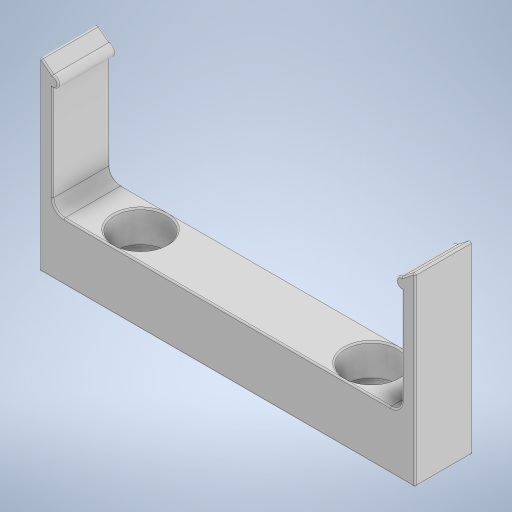
# Autodesk Inventor part: Top bot holder
Saved by Autodesk Inventor 2024 (Build 280153000, 153)
## iProperties
Created: 2024-04-04
Part Number: Top bot holder
Material: Generic
Document SubType Name: Modeling
Designer: jens1
Density: 1 g/cm^3
Appearance: Default
Author: jens1
## iProperties of the stored document Top bot holder_3DPrint.ipt
Created: 2024-04-04
Part Number: Top bot holder_3DPrint
Material: Generic
Document SubType Name: Modeling
Designer: jens1
Density: 1 g/cm^3
Appearance: Default
Author: jens1
Autodesk Inventor part; units mm, degrees
ref_plane "YZ Plane" through (0, 0, 0) normal (1, 0, 0) x (0, 1, 0)
ref_plane "XZ Plane" through (0, 0, 0) normal (0, 1, 0) x (-1, 0, 0)
ref_plane "XY Plane" through (0, 0, 0) normal (0, 0, 1) x (1, 0, 0)
sketch "Sketch1" plane through (0, 0, 0) normal (0, 0, 1) x (1, 0, 0)
  line L0 (0, 0) -> (65, 0)
  line L1 (65, 0) -> (65, 10)
  line L2 (65, 10) -> (0, 10)
  line L3 (0, 10) -> (0, 0)
  line L4 (0, 10) -> (2.25, 10)
  line L5 (2.25, 10) -> (2.25, 30.5)
  line L6 (2.25, 30.5) -> (0, 30.5)
  line L7 (0, 30.5) -> (0, 10)
  circle A0 centre (2.25, 29.5) radius 1
  line L8 (65, 10) -> (62.75, 10)
  line L9 (62.75, 10) -> (62.75, 30.5)
  line L10 (62.75, 30.5) -> (65, 30.5)
  line L11 (65, 30.5) -> (65, 10)
  circle A1 centre (62.75, 29.5) radius 1
  line L12 (0, 30.5) -> (2.25, 30.5)
  line L13 (2.25, 30.5) -> (2.25, 32.25)
  line L14 (2.25, 32.25) -> (0, 32.25)
  line L15 (0, 32.25) -> (0, 30.5)
  line L16 (62.75, 30.5) -> (65, 30.5)
  line L17 (65, 30.5) -> (65, 32.25)
  line L18 (65, 32.25) -> (62.75, 32.25)
  line L19 (62.75, 32.25) -> (62.75, 30.5)
  line L20 (0, 32.25) -> (2.25, 30.5)
  line L21 (62.75, 30.5) -> (65, 32.25)
  point P0 (62.75, 28.5)
  point P1 (2.25, 10)
  point P2 (2.25, 28.5)
  dimension "d4" = 2
  dimension "d7" = 2
  dimension "d0" = 65
  dimension "d1" = 10
  dimension "d2" = 2.25
  dimension "d3" = 20.5
  dimension "d5" = 2.25
  dimension "d6" = 20.5
  dimension "d31" = 2.25
  dimension "d32" = 1.75
  dimension "d33" = 2.25
  dimension "d34" = 1.75
  constraints: 44 end point, 10 parallel, 5 horizontal, 5 perpendicular, 2 point on line, 6 other
  measures "d0" distance of L2.end L1.end
  measures "d1" distance of L1.end L0.end
  measures "d2" distance of L6.end L5.end
  measures "d3" distance of L5.end L4.end
  measures "d5" distance of L9.end L10.end
  measures "d6" distance of L8.end L9.end
  measures "d31" distance of L14.end L13.end
  measures "d32" distance of L13.end L12.end
  measures "d33" distance of L18.end L17.end
  measures "d34" distance of L16.end L17.end
extrude "Extrusion1" add sketch "Sketch1" along normal blind 10 contours L3 L2 L1 L0 | L7 L6 A0 L5 L2 | L2 L9 A1 L10 L11 | L15 L20 L6 | L10 L21 L17 | A0 L5 | L5 A0 | A1 L9 | L9 A1
fillet "Fillet1" radius 2 2 edges at (2.25, 10, 5) (62.75, 10, 5)
fillet "Fillet2" radius 0.25 2 edges at (0, 32.25, 5) (65, 32.25, 5)
sketch "Sketch2" plane through (4.25, 10, 0) normal (0, 1, 0) x (1, 0, 0)
  line L0 (-4.25, 0) -> (60.75, 0) projected
  line L1 (60.75, 0) -> (60.75, -10) projected
  line L2 (-4.25, -10) -> (60.75, -10) projected
  line L3 (-4.25, 0) -> (-4.25, -10) projected
  point P0 (8.25, -5)
  point P1 (48.25, -5)
  dimension "d12" = 0
  dimension "d13" = 40
  dimension "d14" = 12.5
  dimension "d15" = 5
  measures "d12" vertical distance of point (48.25, -5) point (8.25, -5)
  measures "d13" distance of point (8.25, -5) point (48.25, -5)
  measures "d14" distance from line of L3 point (8.25, -5)
  measures "d15" distance from line of L0 point (48.25, -5)
hole "Hole1" at (12.5, 10, 5) at (52.5, 10, 5) direction (0, -1, 0) diameter 5.5 end through all counterbore diameter 9 counterbore depth 5.5
chamfer "Chamfer1" distance 0.25 angle 45 2 edges at (12.5, 10, 0.5) (52.5, 10, 0.5)
chamfer "Chamfer2" distance 0.25 angle 45 2 edges at (12.5, 4.5, 2.25) (52.5, 4.5, 2.25)
fillet "Fillet3" radius 0.25 26 edges at (0.1402, 31.9634, 10) (1.3267, 31.2181, 10) (0, 15.8694, 10) (2.8358, 10.5858, 10) (32.5, 10, 10) (62.1642, 10.5858, 10) (62.75, 20.25, 10) (2.25, 20.25, 10) (3.25, 29.5, 10) (61.75, 29.5, 10) (64.8598, 31.9634, 10) (65, 15.8694, 10) (63.6733, 31.2181, 10) (64.8598, 31.9634, 0) (65, 15.8694, 0) (63.6733, 31.2181, 0) (61.75, 29.5, 0) (32.5, 10, 0) (2.8358, 10.5858, 0) (2.25, 20.25, 0) (62.75, 20.25, 0) (62.1642, 10.5858, 0) (0.1402, 31.9634, 0) (0, 15.8694, 0) (1.3267, 31.2181, 0) (3.25, 29.5, 0)
fillet "Fillet4" radius 0.25 1 edges at (32.5, 0, 0)
equation "\"d2\" = d5"
equation "\"d34\" = d32"
body "Solid1"
